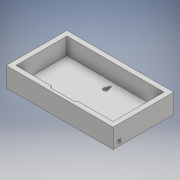
# Autodesk Inventor part: housing
Saved by Autodesk Inventor 2018.2 (Build 222227000, 227)
## iProperties
Created: 2018-03-22
Part Number: housing
Material: Generic
Document SubType Name: Modeling
Designer: wharr
Density: 1 g/cm^3
Appearance: Default
Author: wharr
Autodesk Inventor part; units mm, degrees
ref_plane "YZ Plane" through (0, 0, 0) normal (1, 0, 0) x (0, 1, 0)
ref_plane "XZ Plane" through (0, 0, 0) normal (0, 1, 0) x (-1, 0, 0)
ref_plane "XY Plane" through (0, 0, 0) normal (0, 0, 1) x (1, 0, 0)
sketch "Sketch1" plane through (0, 0, 0) normal (0, 0, 1) x (1, 0, 0)
  line L0 (-100, -52.5) -> (100, -52.5)
  line L1 (100, -52.5) -> (100, 52.5)
  line L2 (100, 52.5) -> (-100, 52.5)
  line L3 (-100, 52.5) -> (-100, -52.5)
  line L4 (-100, -52.5) -> (100, 52.5) construction
  line L5 (100, -52.5) -> (-100, 52.5) construction
  line L6 (-110, 62.5) -> (110, 62.5)
  line L7 (110, 62.5) -> (110, -62.5)
  line L8 (110, -62.5) -> (-110, -62.5)
  line L9 (-110, -62.5) -> (-110, 62.5)
  point P0 (0, 0)
  dimension "d0" = 200
  dimension "d1" = 105
  dimension "d2" = 10
  constraints: 20 end point, 4 parallel, 2 midpoint, 2 perpendicular, 1 horizontal, 3 other
  measures "d0" distance of L1.end L2.end
  measures "d1" distance of L0.end L1.end
  measures "d2" distance between parallel lines of L2 L6
extrude "Extrusion1" add sketch "Sketch1" against normal blind 40
sketch "Sketch2" plane through (-100, 52.5, 0) normal (0, -1, 0) x (1, 0, 0)
  line L0 (200, -40) -> (0, -40) projected
  line L1 (0, 0) -> (0, -40) projected
  line L2 (200, -40) -> (0, -40)
  line L3 (0, -40) -> (0, -35)
  line L4 (0, -35) -> (200, -35)
  line L5 (200, -35) -> (200, -40)
  point P0 (100, 0)
  dimension "d5" = 5
  constraints: 8 end point, 2 parallel, 1 horizontal, 1 perpendicular, 1 point on line
  measures "d5" distance between parallel lines of L0 L4
extrude "Extrusion2" add sketch "Sketch2" along normal up to next
sketch "Sketch3" plane through (0, 0, 0) normal (0, 0, 1) x (1, 0, 0)
  line L0 (100, -52.5) -> (-100, -52.5) projected
  line L1 (0, -52.5) -> (0, -62.5)
  line L2 (110, -62.5) -> (-110, -62.5) projected
  line L3 (-22.5, -56.5) -> (22.5, -56.5)
  line L4 (22.5, -52.5) -> (-22.5, -52.5)
  line L5 (-22.5, -56.5) -> (22.5, -52.5) construction
  line L6 (22.5, -56.5) -> (-22.5, -52.5) construction
  arc A0 (-26.5, -52.5) -> (-22.5, -56.5) centre (-22.5, -52.5) ccw
  arc A1 (22.5, -56.5) -> (26.5, -52.5) centre (22.5, -52.5) ccw
  line L7 (-26.5, -52.5) -> (-22.5, -52.5)
  line L8 (22.5, -52.5) -> (26.5, -52.5)
  point P0 (0, 0)
  point P1 (0, -54.5)
  dimension "d11" = 8
  constraints: 14 end point, 4 midpoint, 4 point on circle, 3 point on line, 2 centre point, 2 coincident, 2 collinear, 1 parallel, 1 perpendicular
  measures "d11" diameter of L3 L0
extrude "Extrusion3" cut sketch "Sketch3" against normal blind 5
sketch "Sketch4" plane through (0, 0, -40) normal (0, 0, -1) x (-1, 0, 0)
  line L0 (110, 62.5) -> (-110, 62.5) projected
  line L1 (0, 62.5) -> (0, -62.5)
  line L2 (-110, -62.5) -> (110, -62.5) projected
  arc A0 (-2.5, 36.8301) -> (2.5, 36.8301) centre (0, 32.5) ccw
  line L3 (0, 32.5) -> (0, 40.5) construction
  line L4 (2.5, 36.8301) -> (2.5, 40.5)
  line L5 (-2.5, 40.5) -> (-2.5, 36.8301)
  arc A1 (2.5, 40.5) -> (-2.5, 40.5) centre (0, 40.5) ccw
  point P0 (0, 0)
  point P1 (0, 36.5)
  dimension "d14" = 10
  dimension "d15" = 5
  dimension "d17" = 30
  dimension "d18" = 8
  constraints: 10 end point, 4 point on circle, 3 midpoint, 2 centre point, 2 point on line, 2 tangent, 1 parallel
  measures "d14" diameter of A0
  measures "d15" diameter of A1
  measures "d17" distance from line of L3.start L0
  measures "d18" distance of L3.end L3.start
extrude "Extrusion4" cut sketch "Sketch4" against normal through all
sketch "Sketch5" plane through (100, -52.5, 0) normal (-1, 0, 0) x (0, 0, 1)
  line L0 (-35, 105) -> (-35, 0) projected
  line L1 (0, 0) -> (-35, 0) projected
  line L2 (-35, 0) -> (-27.5, 0)
  line L3 (-27.5, 0) -> (-27.5, 5)
  line L4 (-27.5, 5) -> (-35, 5)
  line L5 (-35, 5) -> (-35, 0)
  point P0 (0, 52.5)
  dimension "d21" = 7.5
  dimension "d22" = 5
  constraints: 8 end point, 2 parallel, 1 horizontal, 1 perpendicular
  measures "d21" distance of L4.end L3.end
  measures "d22" distance of L3.end L2.end
extrude "Extrusion5" cut sketch "Sketch5" against normal through all
body "Solid1"
